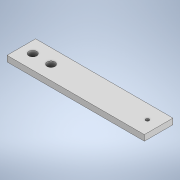
# Autodesk Inventor part: Stationary arm 2
Saved by Autodesk Inventor 2022 (Build 260153000, 153)
## iProperties
Created: 2022-06-15
Part Number: Stationary arm 2
Material: Generic
Document SubType Name: Modeling
Designer: chait
Density: 1 g/cm^3
Appearance: Default
Author: chait
Autodesk Inventor part; units mm, degrees
ref_plane "YZ Plane" through (0, 0, 0) normal (1, 0, 0) x (0, 1, 0)
ref_plane "XZ Plane" through (0, 0, 0) normal (0, 1, 0) x (-1, 0, 0)
ref_plane "XY Plane" through (0, 0, 0) normal (0, 0, 1) x (1, 0, 0)
sketch "Sketch1" plane through (0, 0, 0) normal (0, 1, 0) x (-1, 0, 0)
  line L0 (60, 12.5) -> (-60, 12.5)
  line L1 (-60, 12.5) -> (-60, -12.5)
  line L2 (-60, -12.5) -> (60, -12.5)
  line L3 (60, -12.5) -> (60, 12.5)
  line L4 (60, 12.5) -> (-60, -12.5) construction
  line L5 (-60, 12.5) -> (60, -12.5) construction
  point P0 (0, 0)
  dimension "d0" = 120
  dimension "d1" = 25
  constraints: 12 end point, 2 midpoint, 2 parallel, 1 horizontal, 1 perpendicular
  measures "d0" distance of L2.end L1.end
  measures "d1" distance of L1.end L0.end
extrude "Extrusion1" add sketch "Sketch1" along normal blind 5
sketch "Sketch2" plane through (0, 5, 0) normal (0, 1, 0) x (1, 0, 0)
  circle A0 centre (-50.0145, 0) radius 3.5
  circle A1 centre (-34.0609, 0) radius 3.5
  point P0 (0, 0)
  dimension "d4" = 7
  dimension "d5" = 7
  constraints: 2 centre point
  measures "d4" diameter of A0
  measures "d5" diameter of A1
extrude "Extrusion2" cut sketch "Sketch2" against normal blind 20
sketch "Sketch3" plane through (0, 5, 0) normal (0, 1, 0) x (1, 0, 0)
  circle A0 centre (50.148, 0) radius 1.5
  point P0 (0, 0)
  dimension "d8" = 3
  constraints: 1 centre point
  measures "d8" diameter of A0
extrude "Extrusion3" cut sketch "Sketch3" against normal blind 20
body "Solid1"
